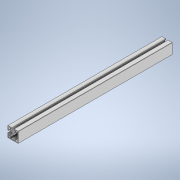
# Autodesk Inventor part: AFST-2020-4-1000
Saved by Autodesk Inventor 2021.1 (Build 251245010, 245A)
## iProperties
Created: 2016-10-06
Part Number: AFST-2020-4-1000
Material: 一般
Document SubType Name: Modeling
Designer: gisen
Density: 1 g/cm^3
Appearance: 既定
Sending System: Autodesk Inventor 2014
Preprocessor: ST-DEVELOPER v15.2
Title: C:\Users\AMS43\Documents\Inventor\AMS\misumi\フレーム_ipt\フレーム_stp\AFST-2020-4.ipt.stp
Author: AMS43
Autodesk Inventor part; units mm, degrees
ref_plane "YZ Plane" through (0, 0, 0) normal (1, 0, 0) x (0, 1, 0)
ref_plane "XZ Plane" through (0, 0, 0) normal (0, 1, 0) x (-1, 0, 0)
ref_plane "作業平面1" through (-9.5, -10, 1000) normal (0, 0, 1) x (1, 0, 0)
sketch "スケッチ1" plane through (-9.5, -10, 1000) normal (0, 0, 1) x (1, 0, 0)
  line L0 (7.35, 18.5) -> (7.35, 20) projected
  line L1 (7.35, 20) -> (0, 20) projected
  arc A0 (0, 20) -> (-0.5, 19.5) centre (0, 19.5) ccw projected
  line L2 (-0.5, 19.5) -> (-0.5, 12.15) projected
  line L3 (-0.5, 12.15) -> (1, 12.15) projected
  line L4 (1, 12.15) -> (1, 14.15) projected
  line L5 (1, 14.15) -> (4.7, 14.15) projected
  line L6 (4.7, 14.15) -> (4.7, 12.15) projected
  line L7 (4.7, 12.15) -> (6.5, 12.15) projected
  line L8 (6.5, 12.15) -> (6.5, 7.85) projected
  line L9 (6.5, 7.85) -> (4.7, 7.85) projected
  line L10 (4.7, 7.85) -> (4.7, 5.85) projected
  line L11 (4.7, 5.85) -> (1, 5.85) projected
  line L12 (1, 5.85) -> (1, 7.85) projected
  line L13 (1, 7.85) -> (-0.5, 7.85) projected
  line L14 (-0.5, 7.85) -> (-0.5, 0.5) projected
  arc A1 (-0.5, 0.5) -> (0, 0) centre (0, 0.5) ccw projected
  line L15 (0, 0) -> (19, 0) projected
  arc A2 (19, 0) -> (19.5, 0.5) centre (19, 0.5) ccw projected
  line L16 (19.5, 0.5) -> (19.5, 19.5) projected
  arc A3 (19.5, 19.5) -> (19, 20) centre (19, 19.5) ccw projected
  line L17 (19, 20) -> (11.65, 20) projected
  line L18 (11.65, 20) -> (11.65, 18.5) projected
  line L19 (11.65, 18.5) -> (13.65, 18.5) projected
  line L20 (13.65, 18.5) -> (13.65, 14.8) projected
  line L21 (13.65, 14.8) -> (11.65, 14.8) projected
  line L22 (11.65, 14.8) -> (11.65, 13) projected
  line L23 (11.65, 13) -> (7.35, 13) projected
  line L24 (7.35, 13) -> (7.35, 14.8) projected
  line L25 (7.35, 14.8) -> (5.35, 14.8) projected
  line L26 (5.35, 14.8) -> (5.35, 18.5) projected
  line L27 (5.35, 18.5) -> (7.35, 18.5) projected
  arc A4 (17.7174, 15.4132) -> (17.6402, 15.0252) centre (17.9, 15.1752) ccw projected
  line L28 (17.6402, 15.0252) -> (17.9598, 14.4715) projected
  arc A5 (18, 14.3215) -> (17.9598, 14.4715) centre (17.7, 14.3215) ccw projected
  line L29 (18, 14.3215) -> (18, 6.7162) projected
  arc A6 (17.7225, 6.4162) -> (18, 6.7162) centre (17.7, 6.7153) ccw projected
  line L30 (17.7225, 6.4162) -> (17.0355, 6.4162) projected
  arc A7 (17.0355, 6.4162) -> (16.8233, 6.3283) centre (17.0355, 6.1162) ccw projected
  line L31 (16.8233, 6.3283) -> (15.9875, 5.4924) projected
  arc A8 (15.9875, 5.4924) -> (16.2388, 4.9829) centre (16.1996, 5.2803) ccw projected
  arc A9 (14.5171, 3.2612) -> (16.2388, 4.9829) centre (16.5, 3) ccw projected
  arc A10 (14.5171, 3.2612) -> (14.2973, 3.5902) centre (14.2197, 3.3004) ccw projected
  line L32 (14.2973, 3.5902) -> (14.2135, 3.6127) projected
  arc A11 (14.2135, 3.6127) -> (13.9237, 3.535) centre (14.1359, 3.3229) ccw projected
  line L33 (13.9237, 3.535) -> (13.0879, 2.6991) projected
  arc A12 (13.0879, 2.6991) -> (13, 2.487) centre (13.3, 2.487) ccw projected
  line L34 (13, 2.487) -> (13, 1.8) projected
  arc A13 (12.7, 1.5) -> (13, 1.8) centre (12.7, 1.8) ccw projected
  line L35 (12.7, 1.5) -> (5.1785, 1.5) projected
  arc A14 (5.0285, 1.5402) -> (5.1785, 1.5) centre (5.1785, 1.8) ccw projected
  line L36 (5.0285, 1.5402) -> (4.4748, 1.8598) projected
  arc A15 (4.4748, 1.8598) -> (4.0868, 1.7826) centre (4.3248, 1.6) ccw projected
  arc A16 (4.0868, 4.2174) -> (4.0868, 1.7826) centre (2.5, 3) ccw projected
  arc A17 (4.0868, 4.2174) -> (4.4748, 4.1402) centre (4.3248, 4.4) ccw projected
  line L37 (4.4748, 4.1402) -> (6.2409, 5.1598) projected
  arc A18 (6.3909, 5.2) -> (6.2409, 5.1598) centre (6.3909, 4.9) ccw projected
  line L38 (6.3909, 5.2) -> (7.05, 5.2) projected
  arc A19 (7.05, 5.2) -> (7.35, 5.5) centre (7.05, 5.5) ccw projected
  line L39 (7.35, 5.5) -> (7.35, 6.4) projected
  arc A20 (7.95, 7) -> (7.35, 6.4) centre (7.95, 6.4) ccw projected
  line L40 (7.95, 7) -> (9.2042, 7) projected
  arc A21 (9.2042, 7) -> (9.4163, 7.0879) centre (9.2042, 7.3) ccw projected
  line L41 (9.4163, 7.0879) -> (9.9752, 7.6468) projected
  arc A22 (9.9752, 7.6468) -> (10.0529, 7.9366) centre (9.7631, 7.8589) ccw projected
  line L42 (10.0529, 7.9366) -> (9.9987, 8.1389) projected
  arc A23 (9.9987, 8.1389) -> (9.6768, 8.3595) centre (9.7089, 8.0612) ccw projected
  arc A24 (11.1405, 9.8232) -> (9.6768, 8.3595) centre (9.5, 10) ccw projected
  arc A25 (11.1405, 9.8232) -> (11.3611, 9.5013) centre (11.4388, 9.7911) ccw projected
  line L43 (11.3611, 9.5013) -> (11.5634, 9.4471) projected
  arc A26 (11.5634, 9.4471) -> (11.8532, 9.5248) centre (11.6411, 9.7369) ccw projected
  line L44 (11.8532, 9.5248) -> (12.4121, 10.0837) projected
  arc A27 (12.4121, 10.0837) -> (12.5, 10.2958) centre (12.2, 10.2958) ccw projected
  line L45 (12.5, 10.2958) -> (12.5, 11.55) projected
  arc A28 (13.1, 12.15) -> (12.5, 11.55) centre (13.1, 11.55) ccw projected
  line L46 (13.1, 12.15) -> (14, 12.15) projected
  arc A29 (14, 12.15) -> (14.2652, 12.4701) centre (13.966, 12.4481) ccw projected
  line L47 (14.2652, 12.4701) -> (14.2652, 13.0488) projected
  arc A30 (14.3054, 13.1988) -> (14.2652, 13.0488) centre (14.5652, 13.0488) ccw projected
  line L48 (14.3054, 13.1988) -> (15.3598, 15.0252) projected
  arc A31 (15.3598, 15.0252) -> (15.2826, 15.4132) centre (15.1, 15.1752) ccw projected
  arc A32 (17.7174, 15.4132) -> (15.2826, 15.4132) centre (16.5, 17) ccw projected
  circle A33 centre (2.5, 17) radius 2 projected
  point P0 (9.5, 10)
extrude "押し出し1" add sketch "スケッチ1" along normal blind 290
